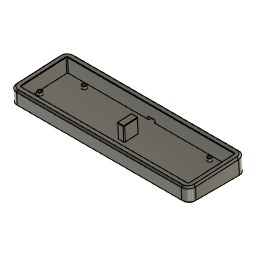
Tsuru MFR2 (Autodesk Fusion 360 design; units mm, degrees)
Autodesk Fusion 360 part; units mm, degrees
sketch "Outline Sketch" plane through (0, 0, 0) normal (0, 0, 1) x (1, 0, 0)
  line L0 (107.2768, 73.5265) -> (316.8268, 73.5265) construction
  line L1 (316.8268, 73.5265) -> (316.8268, 16.3765) construction
  line L2 (316.8268, 16.3765) -> (107.2768, 16.3765) construction
  line L3 (107.2768, 16.3765) -> (107.2768, 73.5265) construction
  line L4 (317.3268, 15.8765) -> (106.7768, 15.8765)
  line L5 (106.7768, 15.8765) -> (106.7768, 74.0265)
  line L6 (106.7768, 74.0265) -> (317.3268, 74.0265)
  line L7 (317.3268, 74.0265) -> (317.3268, 15.8765)
  line L8 (324.3268, 8.8765) -> (99.7768, 8.8765)
  line L9 (99.7768, 8.8765) -> (99.7768, 81.0265)
  line L10 (99.7768, 81.0265) -> (324.3268, 81.0265)
  line L11 (324.3268, 81.0265) -> (324.3268, 8.8765)
  dimension "d1" = 209.55
  dimension "d2" = 57.15
  dimension "d3" = -0.5
  dimension "d4" = -7.5
  constraint horizontal L0
  constraint vertical L1
  constraint horizontal L2
  constraint vertical L3
  measures "d1" distance of L0.start L0.end
  measures "d2" distance of L0.start L2.end
extrude "Extrude1" add sketch "Outline Sketch" along normal blind 18.06
sketch "Angle Sketch" plane through (324.3268, 0, 0) normal (1, 0, 0) x (0, 1, 0)
  line L0 (8.8765, 0) -> (81.0265, 0)
  line L1 (81.0265, 0) -> (81.0265, 18.06)
  line L2 (81.0265, 18.06) -> (8.8765, 18.06)
  line L3 (8.8765, 18.06) -> (8.8765, 0)
  line L4 (8.8765, 18.06) -> (8.8765, -0.215)
  line L5 (8.8765, -0.215) -> (108.7394, -5.4486)
  line L6 (8.8765, -0.215) -> (108.8765, -0.215) construction
  dimension "d7" = 18.275
  dimension "d8" = 100
  dimension "d9" = 3
  constraint coincident L2.end L3.start
  constraint perpendicular L0 L4
  constraint horizontal L6
  measures "d7" distance of L2.end L4.end
  measures "d8" distance of L4.end L5.end
  measures "d9" angle of L5 L6
ref_plane "WorkPlane1" through (324.3268, 58.8079, -2.8318) normal (0, -0.052336, -0.99863) x (0, 0.99863, -0.052336)
sketch "Bottom Sketch for Angle" plane through (0, 0, 0) normal (0, 0, -1) x (1, 0, 0)
  line L0 (317.3268, -74.0265) -> (106.7768, -74.0265)
  line L1 (106.7768, -74.0265) -> (106.7768, -15.8765)
  line L2 (106.7768, -15.8765) -> (317.3268, -15.8765)
  line L3 (317.3268, -15.8765) -> (317.3268, -74.0265)
  line L4 (99.7768, -81.0265) -> (324.3268, -81.0265)
  line L5 (324.3268, -81.0265) -> (324.3268, -8.8765)
  line L6 (324.3268, -8.8765) -> (99.7768, -8.8765)
  line L7 (99.7768, -8.8765) -> (99.7768, -81.0265)
  line L8 (99.7768, -81.0265) -> (324.3268, -81.0265)
  line L9 (324.3268, -81.0265) -> (324.3268, -8.8765)
  line L10 (324.3268, -8.8765) -> (99.7768, -8.8765)
  line L11 (99.7768, -8.8765) -> (99.7768, -81.0265)
  constraint horizontal L8
  constraint vertical L9
  constraint horizontal L10
  constraint vertical L11
  constraint coincident L5.end L6.start
  constraint coincident L4.start L7.end
extrude "Extrude2" add sketch "Bottom Sketch for Angle" along normal up to surface contours L0 L1 L2 L3 | L4 L5 L6 L7 L8 L9 L10 L11 end surface through (324.3268, 58.8079, -2.8318) normal (0, -0.052336, -0.99863) offset 0
sketch "USB C Hole Internal Sketch" plane through (0, 74.0265, 0) normal (0, -1, 0) x (1, 0, 0)
  line L0 (106.7768, 0) -> (317.3268, 0)
  line L1 (317.3268, 0) -> (317.3268, 18.06)
  line L2 (317.3268, 18.06) -> (106.7768, 18.06)
  line L3 (106.7768, 18.06) -> (106.7768, 0)
  line L4 (107.2768, 18.06) -> (107.2768, 0) construction
  line L5 (107.2768, 0) -> (212.0518, 0) construction
  line L6 (212.0518, 0) -> (212.0518, 1.83) construction
  line L7 (216.7768, 3.66) -> (207.3268, 3.66)
  line L8 (207.3268, 3.66) -> (207.3268, 0)
  line L9 (207.3268, 0) -> (216.7768, 0)
  line L10 (216.7768, 0) -> (216.7768, 3.66)
  line L11 (216.7768, 3.66) -> (207.3268, 0) construction
  line L12 (207.3268, 3.66) -> (216.7768, 0) construction
  point P0 (212.0518, 1.83)
  dimension "d13" = -0.5
  dimension "d14" = 104.775
  dimension "d15" = 1.83
  dimension "d16" = 9.45
  dimension "d17" = 3.66
  constraint perpendicular L4 L5
  constraint perpendicular L5 L6
  constraint horizontal L7
  constraint perpendicular L7 L8
  constraint parallel L7 L9
  constraint parallel L8 L10
  constraint coincident L11 P0
  constraint coincident L12 P0
  constraint coincident P0 L6.end
  measures "d14" distance of L4.end L5.end
  measures "d15" distance of L5.end P0
  measures "d16" distance of L8.end L9.end
  measures "d17" distance of L7.end L8.end
extrude "Extrude3" cut sketch "USB C Hole Internal Sketch" against normal blind 40 contours L0 L7 L8 L9 L10
sketch "USB C Hole External Sketch" plane through (0, 81.0265, 0) normal (0, 1, 0) x (-1, 0, 0)
  line L0 (-216.7768, 3.66) -> (-207.3268, 3.66)
  line L1 (-207.3268, 3.66) -> (-207.3268, 0)
  line L2 (-207.3268, 0) -> (-216.7768, 0)
  line L3 (-216.7768, 0) -> (-216.7768, 3.66)
  line L4 (-99.7768, -3.9962) -> (-99.7768, 18.06)
  line L5 (-99.7768, 18.06) -> (-324.3268, 18.06)
  line L6 (-324.3268, 18.06) -> (-324.3268, -3.9962)
  line L7 (-324.3268, -3.9962) -> (-99.7768, -3.9962)
  line L8 (-216.7768, 3.66) -> (-207.3268, 0) construction
  line L9 (-207.3268, 3.66) -> (-216.7768, 0) construction
  circle A0 centre (-212.0518, 1.83) radius 0.3011 construction
  line L10 (-205.0768, 5.91) -> (-219.0268, 5.91)
  line L11 (-219.0268, 5.91) -> (-219.0268, -2.25)
  line L12 (-219.0268, -2.25) -> (-205.0768, -2.25)
  line L13 (-205.0768, -2.25) -> (-205.0768, 5.91)
  line L14 (-205.0768, 5.91) -> (-219.0268, -2.25) construction
  line L15 (-219.0268, 5.91) -> (-205.0768, -2.25) construction
  point P0 (-212.0518, 1.83)
  dimension "d20" = 13.95
  dimension "d21" = 8.16
  constraint coincident L0.start L3.end
  constraint coincident L1.end L2.start
  constraint coincident L0.end L1.start
  constraint coincident L2.end L3.start
  constraint midpoint L9 P0
  constraint horizontal L10
  constraint perpendicular L10 L11
  constraint parallel L10 L12
  constraint parallel L11 L13
  constraint coincident L14 P0
  constraint coincident L15 P0
  constraint coincident P0 A0.centre
  measures "d20" distance of L11.end L12.end
  measures "d21" distance of L10.end L11.end
extrude "Extrude4" cut sketch "USB C Hole External Sketch" against normal blind 4 contours L10 L11 L12 L13
sketch "Screw Post and Center Blocker Sketch" plane through (0, 0, 0) normal (0, 0, 1) x (-1, 0, 0)
  line L0 (-216.7768, -77.0265) -> (-207.3268, -77.0265)
  line L1 (-207.3268, -77.0265) -> (-207.3268, -74.0265)
  line L2 (-207.3268, -74.0265) -> (-106.7768, -74.0265)
  line L3 (-106.7768, -74.0265) -> (-106.7768, -15.8765)
  line L4 (-106.7768, -15.8765) -> (-317.3268, -15.8765)
  line L5 (-317.3268, -15.8765) -> (-317.3268, -74.0265)
  line L6 (-317.3268, -74.0265) -> (-216.7768, -74.0265)
  line L7 (-216.7768, -74.0265) -> (-216.7768, -77.0265)
  line L8 (-316.8268, -73.5265) -> (-216.2768, -73.5265) construction
  line L9 (-216.2768, -73.5265) -> (-216.2768, -76.5265) construction
  line L10 (-216.2768, -76.5265) -> (-207.8268, -76.5265) construction
  line L11 (-207.8268, -76.5265) -> (-207.8268, -73.5265) construction
  line L12 (-207.8268, -73.5265) -> (-107.2768, -73.5265) construction
  line L13 (-107.2768, -73.5265) -> (-107.2768, -16.3765) construction
  line L14 (-107.2768, -16.3765) -> (-316.8268, -16.3765) construction
  line L15 (-316.8268, -16.3765) -> (-316.8268, -73.5265) construction
  circle A0 centre (-110.8488, -35.4265) radius 2.75
  circle A1 centre (-133.4708, -68.4665) radius 2.75
  circle A2 centre (-290.6328, -68.4665) radius 2.75
  circle A3 centre (-313.2548, -35.4265) radius 2.75
  line L16 (-107.2768, -73.5265) -> (-316.8268, -16.3765) construction
  line L17 (-316.8268, -73.5265) -> (-107.2768, -16.3765) construction
  circle A4 centre (-212.0518, -44.9515) radius 1.922 construction
  line L18 (-216.8143, -54.4765) -> (-207.2893, -54.4765) construction
  line L19 (-207.2893, -54.4765) -> (-207.2893, -35.4265) construction
  line L20 (-207.2893, -35.4265) -> (-216.8143, -35.4265) construction
  line L21 (-216.8143, -35.4265) -> (-216.8143, -54.4765) construction
  line L22 (-216.8143, -54.4765) -> (-207.2893, -35.4265) construction
  line L23 (-207.2893, -54.4765) -> (-216.8143, -35.4265) construction
  line L24 (-216.3143, -35.9265) -> (-216.3143, -53.9765)
  line L25 (-216.3143, -53.9765) -> (-207.7893, -53.9765)
  line L26 (-207.7893, -53.9765) -> (-207.7893, -35.9265)
  line L27 (-207.7893, -35.9265) -> (-216.3143, -35.9265)
  point P0 (-212.0518, -44.9515)
  dimension "d24" = -0.5
  dimension "d25" = 5.5
  dimension "d26" = 19.05
  dimension "d27" = 3.572
  dimension "d28" = 5.5
  dimension "d29" = 26.194
  dimension "d30" = 5.06
  dimension "d31" = 5.5
  dimension "d32" = 5.5
  dimension "d33" = 26.194
  dimension "d34" = 5.06
  dimension "d35" = 19.05
  dimension "d36" = 3.572
  dimension "d37" = 9.525
  dimension "d38" = 19.05
  dimension "d39" = -0.5
  constraint midpoint L17 P0
  constraint horizontal L18
  constraint perpendicular L18 L19
  constraint parallel L18 L20
  constraint parallel L19 L21
  constraint coincident L22 P0
  constraint coincident L23 P0
  constraint coincident P0 A4.centre
  measures "d25" diameter of A0
  measures "d26" distance of L14 A0.centre
  measures "d27" distance of L13 A0.centre
  measures "d28" diameter of A1
  measures "d29" distance of L13 A1.centre
  measures "d30" distance of L12 A1.centre
  measures "d31" diameter of A2
  measures "d32" diameter of A3
  measures "d33" distance of L15 A2.centre
  measures "d34" distance of L8 A2.centre
  measures "d35" distance of L14 A3.centre
  measures "d36" distance of L15 A3.centre
  measures "d37" distance of L19.end L20.end
  measures "d38" distance of L18.end L19.end
extrude "Extrude5" add sketch "Screw Post and Center Blocker Sketch" along normal blind 18.06 contours L24 L25 L26 L27
extrude "Extrude6" add sketch "Screw Post and Center Blocker Sketch" along normal blind 3.46 contours A0 | A1 | A2 | A3
hole "Hole1" at (133.4708, 68.4665, 3.46) direction (0, 0, -1) diameter 3.2 depth 4 tip angle 180
hole "Hole2" at (110.8488, 35.4265, 3.46) direction (0, 0, -1) diameter 3.2 depth 4 tip angle 180
hole "Hole3" at (290.6328, 68.4665, 3.46) direction (0, 0, -1) diameter 3.2 depth 4 tip angle 180
hole "Hole4" at (313.2548, 35.4265, 3.46) direction (0, 0, -1) diameter 3.2 depth 4 tip angle 180
fillet "Fillet1" radius 1.55 4 edges at (216.7768, 75.5265, 3.66) (216.7768, 75.5265, 0) (207.3268, 75.5265, 0) (207.3268, 75.5265, 3.66)
fillet "Fillet2" radius 3.8 4 edges at (219.0268, 79.0265, 5.91) (219.0268, 79.0265, -2.25) (205.0768, 79.0265, -2.25) (205.0768, 79.0265, 5.91)
chamfer "Chamfer1" distance 0.25 angle 45 8 edges at (212.0518, 81.0265, 5.91) (206.1898, 81.0265, 4.797) (205.0768, 81.0265, 1.83) (206.1898, 81.0265, -1.137) (212.0518, 81.0265, -2.25) (217.9138, 81.0265, -1.137) (219.0268, 81.0265, 1.83) (217.9138, 81.0265, 4.797)
fillet "Fillet3" radius 9 4 edges at (324.3268, 81.0265, 7.0319) (324.3268, 8.8765, 8.9225) (99.7768, 8.8765, 8.9225) (99.7768, 81.0265, 7.0319)
fillet "Fillet4" radius 1 8 edges at (106.7768, 74.0265, 9.03) (106.7768, 15.8765, 9.03) (317.3268, 74.0265, 9.03) (317.3268, 15.8765, 9.03) (216.3143, 53.9765, 9.03) (207.7893, 53.9765, 9.03) (207.7893, 35.9265, 9.03) (216.3143, 35.9265, 9.03)
chamfer "Chamfer2" distance 2 angle 45 16 edges at (99.7768, 44.9515, 18.06) (102.4128, 11.5125, 18.06) (212.0518, 8.8765, 18.06) (321.6907, 11.5125, 18.06) (324.3268, 44.9515, 18.06) (321.6907, 78.3904, 18.06) (212.0518, 81.0265, 18.06) (102.4128, 78.3904, 18.06) (99.7768, 44.9515, -2.1056) (102.4128, 11.5125, -0.3531) (212.0518, 8.8765, -0.215) (321.6907, 11.5125, -0.3531) (324.3268, 44.9515, -2.1056) (321.6907, 78.3904, -3.8581) (212.0518, 81.0265, -3.9962) (102.4128, 78.3904, -3.8581)
chamfer "Chamfer3" distance 0.5 angle 45 8 edges at (212.0518, 74.0265, 18.06) (317.0339, 73.7336, 18.06) (317.3268, 44.9515, 18.06) (317.0339, 16.1694, 18.06) (212.0518, 15.8765, 18.06) (107.0697, 16.1694, 18.06) (106.7768, 44.9515, 18.06) (107.0697, 73.7336, 18.06)
chamfer "Chamfer4" distance 0.5 angle 45 8 edges at (207.7893, 44.9515, 18.06) (208.0822, 36.2194, 18.06) (212.0518, 35.9265, 18.06) (216.0214, 36.2194, 18.06) (216.3143, 44.9515, 18.06) (216.0214, 53.6836, 18.06) (212.0518, 53.9765, 18.06) (208.0822, 53.6836, 18.06)
extrude "Extrude7" add 1 faces at (246.4768, 56.3107, -2.7009) along direction (0, 0.052336, 0.99863) blind 1
move_body "Move1" bodies 1 to x (1, 0, 0) y (0, 0.99863, 0.052336) z (0, -0.052336, 0.99863) at (0, -0.0018, -0.5695)
equation "d1 = 19.05 mm * 11"
equation "d2 = 19.05 mm * 3"
equation "d33 = d29"
equation "d34 = d30"
equation "d35 = d26"
equation "d36 = d27"
